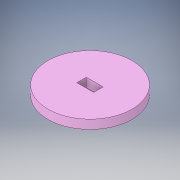
# Autodesk Inventor part: HOMBRO_SOST.EJE
Saved by Autodesk Inventor 2019 (Build 230136000, 136)
## iProperties
Created: 2020-02-12
Part Number: HOMBRO_SOST.EJE
Material: Genérico
Document SubType Name: Modeling
Designer: omar-
Density: 1 g/cm^3
Appearance: Valor por defecto
Author: omar-
Autodesk Inventor part; units mm, degrees
ref_plane "YZ Plane" through (0, 0, 0) normal (1, 0, 0) x (0, 1, 0)
ref_plane "XZ Plane" through (0, 0, 0) normal (0, 1, 0) x (-1, 0, 0)
ref_plane "XY Plane" through (0, 0, 0) normal (0, 0, 1) x (1, 0, 0)
sketch "Boceto1" plane through (0, 0, 0) normal (0, 1, 0) x (-1, 0, 0)
  line L0 (-3, 1.69) -> (3, 1.69)
  line L1 (3, 1.69) -> (3, -1.69)
  line L2 (3, -1.69) -> (-3, -1.69)
  line L3 (-3, -1.69) -> (-3, 1.69)
  line L4 (-3, 1.69) -> (3, -1.69) construction
  line L5 (3, 1.69) -> (-3, -1.69) construction
  circle A0 centre (0, 0) radius 15
  dimension "d0" = 6
  dimension "d1" = 3.38
  dimension "d2" = 30
  constraints: 12 end point, 2 midpoint, 2 parallel, 1 centre point, 1 coincident, 1 horizontal, 1 perpendicular
  measures "d0" distance of L1.end L2.end
  measures "d1" distance of L0.end L1.end
  measures "d2" diameter of A0
extrude "Extrusión1" add sketch "Boceto1" along normal blind 3.18
